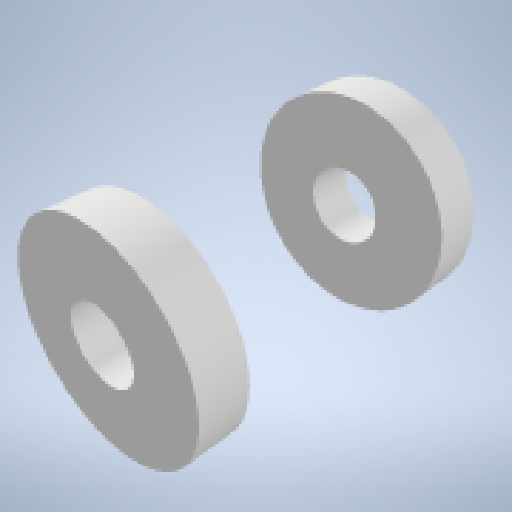
# Autodesk Inventor part: moving piece
Saved by Autodesk Inventor 2025 (Build 290162000, 162)
## iProperties
Created: 2025-01-09
Part Number: moving piece
Material: Generic
Document SubType Name: Modeling
Designer: 5014070
Density: 1 g/cm^3
Appearance: Default
Author: 5014070
Autodesk Inventor part; units mm, degrees
ref_plane "YZ Plane" through (0, 0, 0) normal (1, 0, 0) x (0, 1, 0)
ref_plane "XZ Plane" through (0, 0, 0) normal (0, 1, 0) x (-1, 0, 0)
ref_plane "XY Plane" through (0, 0, 0) normal (0, 0, 1) x (1, 0, 0)
sketch "Sketch1" plane through (0, 0, 0) normal (0, 0, 1) x (1, 0, 0)
  circle A0 centre (0, 0) radius 4
  circle A1 centre (0, 0) radius 11.43
  dimension "d0" = 8
  dimension "d1" = 22.86
  constraints: 2 centre point, 2 coincident
  measures "d0" diameter of A0
  measures "d1" diameter of A1
extrude "Extrusion1" add sketch "Sketch1" along normal blind 5.08 and the other way blind 29.21
extrude "Extrusion2" cut sketch "Sketch1" against normal blind 24.13
body "Solid1"
